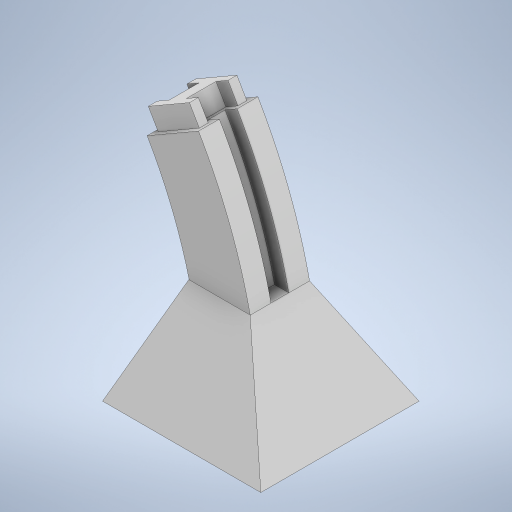
# Autodesk Inventor part: LightRail_endSection
Saved by Autodesk Inventor 2023 (Build 270158000, 158)
## iProperties
Created: 2023-04-11
Part Number: LightRail_endSection
Material: Generic
Document SubType Name: Modeling
Designer: ringl
Density: 1 g/cm^3
Appearance: Default
Author: ringl
Autodesk Inventor part; units mm, degrees
sketch "Sketch2" plane through (0, 0, 0) normal (0, 1, 0) x (-1, 0, 0)
  line L0 (15, 15) -> (-15, 15)
  line L1 (-15, -15) -> (15, -15)
  line L2 (15, 4.5) -> (8, 4.5)
  line L3 (8, 4.5) -> (8, -4.5)
  line L4 (8, -4.5) -> (15, -4.5)
  line L5 (-15, 4.5) -> (-8, 4.5)
  line L6 (-8, 4.5) -> (-8, -4.5)
  line L7 (-8, -4.5) -> (-15, -4.5)
  line L8 (15, -15) -> (15, -4.5)
  line L9 (15, 4.5) -> (15, 15)
  line L10 (-15, 15) -> (-15, 4.5)
  line L11 (-15, -4.5) -> (-15, -15)
  point P0 (0, 0)
  dimension "d18" = 9
  dimension "d19" = 7
  dimension "d21" = 16
  dimension "d22" = 30
  dimension "d23" = 15
  dimension "d24" = 4.5
  dimension "d25" = 8
  constraints: 24 end point, 7 parallel, 4 perpendicular, 3 equal length, 3 horizontal, 2 point on line
  measures "d18" distance of L5.end L6.end
  measures "d19" distance of L5.start L5.end
  measures "d21" distance between parallel lines of L3 L6
  measures "d22" distance between parallel lines of L1 L0
  measures "d23" distance from line of L1 point (0, 0)
  measures "d24" distance from line of point (0, 0) L5
  measures "d25" distance from line of L6 point (0, 0)
sketch "Sketch6" plane through (0, 0, 0) normal (0, 0, 1) x (1, 0, 0)
  arc A0 (0, 0) -> (-110, 190.5256) centre (-220, 0) ccw
  line L0 (-220, 0) -> (-110, 190.5256) construction
  line L1 (-220, 0) -> (0, 0) construction
  dimension "d41" = 220
  dimension "d42" = 60
  dimension "d43" = 220
  dimension "d44" = 0
  constraints: 4 end point, 2 point on circle, 1 centre point, 1 horizontal
  measures "d41" radius of A0
  measures "d42" angle of L1 L0
  measures "d43" distance of L0.start point (0, 0)
  measures "d44" distance of L1.end point (0, 0)
sweep "Sweep2" add profiles "Sketch2" path "Sketch6"
sketch "Sketch7" plane through (-102.5, 203.516, 4.5) normal (-0.8660254, 0.5, 0) x (0, 0, 1)
  line L0 (-16.5, -3) -> (-12, -3)
  line L1 (-12, -3) -> (-12, -10)
  line L2 (-12, -10) -> (3, -10)
  line L3 (3, -10) -> (3, -3)
  line L4 (3, -3) -> (7.5, -3)
  line L5 (7.5, -3) -> (7.5, -27)
  line L6 (7.5, -27) -> (3, -27)
  line L7 (3, -27) -> (3, -20)
  line L8 (3, -20) -> (-12, -20)
  line L9 (-12, -20) -> (-12, -27)
  line L10 (-12, -27) -> (-16.5, -27)
  line L11 (-16.5, -27) -> (-16.5, -3)
  line L12 (-19.5, 0) -> (-19.5, -30) projected
  line L13 (-9, -7) -> (-9, 0) projected
  line L14 (0, 0) -> (0, -7) projected
  line L15 (10.5, -30) -> (10.5, 0) projected
  line L16 (-19.5, -30) -> (-9, -30) projected
  line L17 (-9, 0) -> (-19.5, 0) projected
  line L18 (0, -30) -> (10.5, -30) projected
  line L19 (-9, -23) -> (0, -23) projected
  line L20 (0, -7) -> (-9, -7) projected
  point P0 (-4.5, -125)
  point P1 (-14.25, 0)
  dimension "d47" = 3
  dimension "d48" = 3
  dimension "d49" = 3
  dimension "d50" = 3
  dimension "d51" = 3
  dimension "d52" = 3
  dimension "d53" = 3
  dimension "d54" = 3
  dimension "d55" = 3
  constraints: 24 end point, 8 perpendicular, 6 point on line, 1 horizontal, 1 midpoint
  measures "d47" distance between parallel lines of L12 L11
  measures "d48" distance between parallel lines of L13 L1
  measures "d49" distance between parallel lines of L14 L3
  measures "d50" distance between parallel lines of L15 L5
  measures "d51" distance between parallel lines of L16 L10
  measures "d52" distance from line of point (-14.25, 0) L0
  measures "d53" distance between parallel lines of L18 L6
  measures "d54" distance between parallel lines of L19 L8
  measures "d55" distance between parallel lines of L20 L2
extrude "Extrusion3" add sketch "Sketch7" along normal blind 10
sketch "Sketch8" plane through (-116, 180.1333, -12) normal (0, 0, -1) x (-0.8660254, 0.5, 0)
  circle A0 centre (5, 12) radius 2
  line L0 (0, 0) -> (10, 0) projected
  line L1 (10, 24) -> (10, 0) projected
  point P0 (-190.5256, -98)
  dimension "d58" = 4
  dimension "d59" = 12
  dimension "d60" = 5
  constraints: 1 centre point
  measures "d58" diameter of A0
  measures "d59" distance from line of L0 A0.centre
  measures "d60" distance from line of A0.centre L1
extrude "Extrusion4" cut sketch "Sketch8" against normal through all
sketch "Sketch9" plane through (0, 0, 0) normal (0, 1, 0) x (-1, 0, 0)
  line L0 (-40, 40) -> (40, 40)
  line L1 (40, 40) -> (40, -40)
  line L2 (40, -40) -> (-40, -40)
  line L3 (-40, -40) -> (-40, 40)
  point P0 (0, 0)
  dimension "d63" = 80
  dimension "d64" = 80
  dimension "d65" = 40
  dimension "d66" = 40
  constraints: 8 end point, 2 parallel, 1 horizontal, 1 perpendicular
  measures "d63" distance of L1.end L2.end
  measures "d64" distance of L0.end L1.end
  measures "d65" distance from line of L3 point (0, 0)
  measures "d66" distance from line of L0 point (0, 0)
ref_plane "Work Plane1" through (0, 50, 0) normal (0, 1, 0) x (-1, 0, 0)
sketch "Sketch10" plane through (0, 50, 0) normal (0, 1, 0) x (-1, 0, 0)
  line L0 (-9.6, 15) -> (21.4, 15)
  line L1 (21.4, 15) -> (21.4, -15)
  line L2 (21.4, -15) -> (-9.6, -15)
  line L3 (-9.6, -15) -> (-9.6, 15)
  point P0 (0, 0)
  dimension "d68" = 30
  dimension "d69" = 9.6
  dimension "d70" = 15
  dimension "d71" = 31
  constraints: 8 end point, 2 parallel, 1 horizontal, 1 perpendicular
  measures "d68" distance of L2.end L0.start
  measures "d69" distance from line of L3 point (0, 0)
  measures "d70" distance from line of point (0, 0) L0
  measures "d71" distance of L1.end L2.end
loft "Loft1" add profiles "Sketch9", "Sketch10"
ref_plane "Work Plane2" through (0, 0, -79) normal (0, 0, 1) x (1, 0, 0)
sketch "Sketch11" plane through (0, 0, -79) normal (0, 0, 1) x (1, 0, 0)
  line L0 (50, -5) -> (-129.034, -5)
  line L1 (-129.034, -5) -> (-129.034, 135)
  line L2 (-129.034, 135) -> (-90, 202.6089)
  line L3 (-90, 202.6089) -> (50, 95)
  line L4 (50, -5) -> (50, 95)
  point P0 (0, 0)
  dimension "d77" = 100
  dimension "d79" = 140
  dimension "d80" = 67.6089
  dimension "d81" = 140
  dimension "d82" = 150
  dimension "d83" = 50
  dimension "d86" = 5
  constraints: 10 end point, 1 horizontal, 1 perpendicular, 1 vertical
  measures "d77" distance of L0.start L3.end
  measures "d79" distance of L0.end L1.end
  measures "d80" vertical distance of L1.end L2.end
  measures "d81" horizontal distance of L2.end L3.end
  measures "d82" angle of L1 L2
  measures "d83" distance from line of L4 point (0, 0)
  measures "d86" distance from line of point (0, 0) L0
extrude "Extrusion5" [suppressed]
sketch "Sketch12" plane through (-40, 0, 40) normal (0, -1, 0) x (1, 0, 0)
  line L0 (70, -70) -> (10, -70)
  line L1 (10, -70) -> (10, -10)
  line L2 (10, -10) -> (70, -10)
  line L3 (70, -10) -> (70, -70)
  line L4 (0, 0) -> (0, -80) projected
  line L5 (0, -80) -> (80, -80) projected
  line L6 (80, -80) -> (80, 0) projected
  line L7 (80, 0) -> (0, 0) projected
  point P0 (40, -40)
  dimension "d87" = 10
  dimension "d88" = 10
  dimension "d89" = 10
  dimension "d90" = 10
  constraints: 8 end point, 2 parallel, 1 horizontal, 1 perpendicular
  measures "d87" distance between parallel lines of L1 L4
  measures "d88" distance between parallel lines of L5 L0
  measures "d89" distance between parallel lines of L6 L3
  measures "d90" distance between parallel lines of L7 L2
ref_plane "Work Plane3" through (-40, 45, 40) normal (0, -1, 0) x (1, 0, 0)
sketch "Sketch14" plane through (-40, 45, 40) normal (0, -1, 0) x (1, 0, 0)
  line L0 (40.5, -40.5) -> (39.5, -40.5)
  line L1 (39.5, -40.5) -> (39.5, -39.5)
  line L2 (39.5, -39.5) -> (40.5, -39.5)
  line L3 (40.5, -39.5) -> (40.5, -40.5)
  line L4 (80, 0) -> (0, 0) projected
  line L5 (0, 0) -> (0, -80) projected
  point P0 (40, -40)
  point P1 (0, -40)
  dimension "d95" = 1
  dimension "d96" = 1
  dimension "d97" = 39.5
  dimension "d98" = 39.5
  constraints: 8 end point, 2 parallel, 1 horizontal, 1 midpoint, 1 perpendicular
  measures "d95" distance of L1.end L2.end
  measures "d96" distance of L0.end L1.end
  measures "d97" distance between parallel lines of L4 L2
  measures "d98" distance from line of point (0, -40) L1
loft "Loft2" cut profiles "Sketch12", "Sketch14" contours L0 L1 L2 L3 / all
ref_plane "Work Plane4" through (9.6, 50, -45) normal (0, 0, -1) x (-1, 0, 0)
sketch "Sketch15" plane through (9.6, 50, -45) normal (0, 0, -1) x (-1, 0, 0)
  line L0 (-151.4512, 170) -> (229.6, 170)
  line L1 (229.6, 170) -> (229.6, -50)
  line L2 (229.6, -50) -> (-151.4512, 170)
  line L3 (0, 0) -> (7.15, 0) construction
  line L4 (229.6, -50) -> (9.6, -50) construction
  dimension "d105" = 220
  dimension "d107" = 0
  dimension "d108" = 30
  dimension "d109" = 220
  constraints: 9 end point, 1 horizontal, 1 perpendicular
  measures "d105" distance of L1.end L4.end
  measures "d107" vertical distance of L4.end L1.end
  measures "d108" angle of L2 L4
  measures "d109" distance of L0.end L1.end
extrude "Extrusion6" cut sketch "Sketch15" against normal through all
sketch "Sketch16" plane through (-42.4648, 102.5, 15) normal (-0.5, 0.8660254, 0) x (0.8660254, 0.5, 0)
  line L0 (27, 27) -> (27, 22.5)
  line L1 (27, 22.5) -> (20, 22.5)
  line L2 (20, 22.5) -> (20, 7.5)
  line L3 (18.8407, 0) -> (18.8407, 10.5) projected
  line L4 (20, 7.5) -> (27, 7.5)
  line L5 (27, 7.5) -> (27, 3)
  line L6 (27, 3) -> (3, 3)
  line L7 (3, 3) -> (3, 7.5)
  line L8 (3, 7.5) -> (10, 7.5)
  line L9 (10, 7.5) -> (10, 22.5)
  line L10 (10, 22.5) -> (3, 22.5)
  line L11 (3, 22.5) -> (3, 27)
  line L12 (3, 27) -> (27, 27)
  line L13 (30, 30) -> (30, 19.5) projected
  line L14 (30, 19.5) -> (23, 19.5) projected
  line L15 (0, 30) -> (30, 30) projected
  line L16 (23, 19.5) -> (23, 10.5) projected
  line L17 (23, 10.5) -> (30, 10.5) projected
  line L18 (30, 0) -> (0, 0) projected
  line L19 (7, 10.5) -> (7, 19.5) projected
  line L20 (0, 0) -> (0, 10.5) projected
  line L21 (0, 19.5) -> (0, 30) projected
  point P0 (-14.4744, 15)
  dimension "d112" = 3
  dimension "d113" = 3
  dimension "d114" = 3
  dimension "d115" = 3
  dimension "d116" = 3
  dimension "d117" = 3
  dimension "d118" = 3
  dimension "d119" = 3
  dimension "d120" = 3
  constraints: 24 end point, 7 perpendicular, 6 point on line, 1 parallel, 1 vertical
  measures "d112" distance between parallel lines of L13 L0
  measures "d113" distance between parallel lines of L1 L14
  measures "d114" distance between parallel lines of L15 L12
  measures "d115" distance between parallel lines of L16 L2
  measures "d116" distance between parallel lines of L4 L17
  measures "d117" distance between parallel lines of L18 L6
  measures "d118" distance between parallel lines of L19 L9
  measures "d119" distance between parallel lines of L20 L7
  measures "d120" distance between parallel lines of L21 L11
extrude "Extrusion7" add sketch "Sketch16" along normal blind 10
body "Solid2"
